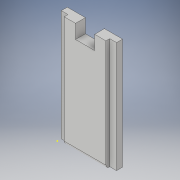
# Autodesk Inventor part: battery_cover
Saved by Autodesk Inventor 2017 (Build 210142000, 142)
## iProperties
Created: 2016-11-20
Part Number: battery_cover
Material: Generic
Document SubType Name: Modeling
Designer: radrajith
Density: 1 g/cm^3
Appearance: Default
Author: radrajith
Autodesk Inventor part; units mm, degrees
ref_plane "YZ Plane" through (0, 0, 0) normal (1, 0, 0) x (0, 1, 0)
ref_plane "XZ Plane" through (0, 0, 0) normal (0, 1, 0) x (-1, 0, 0)
ref_plane "XY Plane" through (0, 0, 0) normal (0, 0, 1) x (1, 0, 0)
sketch "Sketch1" plane through (0, 0, 0) normal (0, 0, 1) x (1, 0, 0)
  line L0 (0, 0) -> (34.8, 0)
  line L1 (34.8, 0) -> (34.8, 69.8)
  line L2 (34.8, 69.8) -> (0, 69.8)
  line L3 (0, 69.8) -> (0, 0)
  line L4 (34.8, 69.8) -> (0, 69.8)
  line L5 (0, 69.8) -> (0, 0)
  line L6 (0, 0) -> (34.8, 0)
  line L7 (34.8, 0) -> (34.8, 69.8)
  dimension "d4" = 34.8
  dimension "d5" = 69.8
  constraints: 16 end point, 4 parallel, 2 horizontal, 2 perpendicular
  measures "d4" distance between parallel lines of L1 L3
  measures "d5" distance between parallel lines of L0 L2
extrude "Extrusion1" add sketch "Sketch1" along normal blind 3.8
sketch "Sketch3" plane through (0, 0, 3.8) normal (0, 0, 1) x (1, 0, 0)
  line L0 (34.8, 69.8) -> (0, 69.8) projected
  line L1 (0, 0) -> (34.8, 0) projected
  line L2 (30.55, 69.8) -> (4.25, 69.8)
  line L3 (4.25, 69.8) -> (4.25, 0)
  line L4 (4.25, 0) -> (30.55, 0)
  line L5 (30.55, 0) -> (30.55, 69.8)
  line L6 (0, 69.8) -> (0, 0) projected
  line L7 (34.8, 0) -> (34.8, 69.8) projected
  dimension "d6" = 26.3
  dimension "d7" = 4.25
  dimension "d8" = 4.25
  constraints: 8 end point, 2 parallel, 2 point on line, 1 horizontal, 1 perpendicular
  measures "d6" distance of L4.end L3.end
  measures "d7" distance between parallel lines of L6 L3
  measures "d8" distance between parallel lines of L7 L5
extrude "Extrusion3" add sketch "Sketch3" along normal blind 2.4 contours L5 L1 L3 L0
sketch "Sketch4" plane through (0, 0, 6.2) normal (0, 0, 1) x (1, 0, 0)
  point P0 (0, 0)
sketch "Sketch5" plane through (0, 0, 6.2) normal (0, 0, 1) x (1, 0, 0)
  line L0 (30.55, 69.8) -> (4.25, 69.8) projected
  line L1 (23.4, 69.8) -> (11.4, 69.8)
  line L2 (11.4, 69.8) -> (11.4, 61)
  line L3 (11.4, 61) -> (23.4, 61)
  line L4 (23.4, 61) -> (23.4, 69.8)
  point P0 (0, 0)
  dimension "d11" = 12
  constraints: 8 end point, 2 parallel, 1 horizontal, 1 perpendicular, 1 point on line
  measures "d11" distance of L3.end L2.end
extrude "Extrusion4" cut sketch "Sketch5" against normal blind 8
fillet "Fillet1" radius 2 1 edges at (17.4, 0, 6.2)
body "Solid1"
